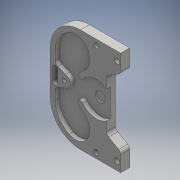
# Autodesk Inventor part: Kompliteringsbit
Saved by Autodesk Inventor 2016 (Build 200138000, 138)
## iProperties
Created: 2017-03-24
Part Number: Kompliteringsbit
Material: Generic
Document SubType Name: Modeling
Designer: 16wise
Density: 1 g/cm^3
Appearance: Default
Author: 16wise
Autodesk Inventor part; units mm, degrees
ref_plane "YZ Plane" through (0, 0, 0) normal (1, 0, 0) x (0, 1, 0)
ref_plane "XZ Plane" through (0, 0, 0) normal (0, 1, 0) x (-1, 0, 0)
ref_plane "XY Plane" through (0, 0, 0) normal (0, 0, 1) x (1, 0, 0)
sketch "Sketch2" plane through (0, 0, 0) normal (0, 1, 0) x (-1, 0, 0)
  line L0 (-51.5, -51.5) -> (51.5, -51.5)
  line L1 (51.5, -51.5) -> (51.5, 51.5)
  line L2 (51.5, 51.5) -> (-51.5, 51.5)
  line L3 (-51.5, 51.5) -> (-51.5, -51.5)
  line L4 (-51.5, -51.5) -> (51.5, 51.5) construction
  line L5 (51.5, -51.5) -> (-51.5, 51.5) construction
  point P0 (0, 0)
  dimension "d6" = 103
  dimension "d7" = 103
  constraints: 12 end point, 2 midpoint, 2 parallel, 1 horizontal, 1 perpendicular
  measures "d6" distance of L2.end L1.end
  measures "d7" distance of L1.end L0.end
extrude "Extrusion2" add sketch "Sketch2" along normal blind 9
fillet "Fillet3" radius 30 1 edges at (-51.5, 4.5, -51.5)
fillet "Fillet4" radius 30 1 edges at (51.5, 4.5, -51.5)
fillet "Fillet5" radius 30 1 edges at (-51.5, 4.5, 51.5)
sketch "Sketch3" plane through (0, 0, 0) normal (0, -1, 0) x (1, 0, 0)
  line L0 (51.5, 51.5) -> (51.5, -21.5) projected
  line L1 (21.5, -51.5) -> (-21.5, -51.5) projected
  line L2 (51.5, 51.5) -> (18.5, 51.5)
  line L3 (18.5, 51.5) -> (18.5, -51.5)
  line L4 (18.5, -51.5) -> (51.5, -51.5)
  line L5 (51.5, -51.5) -> (51.5, 51.5)
  point P0 (0, 0)
  dimension "d13" = 33
  constraints: 8 end point, 2 parallel, 1 horizontal, 1 perpendicular, 1 point on line
  measures "d13" distance of L4.end L3.end
extrude "Extrusion3" cut sketch "Sketch3" against normal blind 9
sketch "Sketch4" plane through (0, 0, 0) normal (0, -1, 0) x (1, 0, 0)
  line L0 (-21.5, 51.5) -> (18.5, 51.5) projected
  line L1 (18.5, 51.5) -> (18.5, 25.5)
  line L2 (18.5, 51.5) -> (18.5, -51.5) projected
  line L3 (18.5, -51.5) -> (18.5, -25.5)
  line L4 (18.5, 25.5) -> (4.5, 25.5)
  line L5 (4.5, 25.5) -> (4.5, -25.5)
  line L6 (4.5, -25.5) -> (18.5, -25.5)
  line L7 (18.5, -25.5) -> (18.5, 25.5)
  point P0 (0, 0)
  dimension "d16" = 26
  dimension "d17" = 26
  dimension "d18" = 14
  constraints: 12 end point, 2 parallel, 2 point on line, 1 horizontal, 1 perpendicular
  measures "d16" distance of L0.end L1.end
  measures "d17" distance of L2.end L3.end
  measures "d18" distance of L6.end L5.end
extrude "Extrusion4" cut sketch "Sketch4" against normal blind 9
sketch "Sketch5" plane through (0, 0, 0) normal (0, -1, 0) x (1, 0, 0)
  line L0 (18.5, 51.5) -> (18.5, 33.5)
  line L1 (18.5, 25.5) -> (18.5, 51.5) projected
  line L2 (4.5, 25.5) -> (4.5, -25.5) projected
  line L3 (18.5, 33.5) -> (4.5, 25.5)
  line L4 (18.5, 25.5) -> (4.5, 25.5) projected
  line L5 (4.5, 25.5) -> (18.5, 25.5)
  line L6 (18.5, 25.5) -> (18.5, 33.5)
  line L7 (18.5, -51.5) -> (-21.5, -51.5) projected
  line L8 (18.5, -51.5) -> (18.5, -33.5)
  line L9 (18.5, -25.5) -> (18.5, -51.5) projected
  line L10 (18.5, -33.5) -> (4.5, -25.5)
  line L11 (4.5, -25.5) -> (18.5, -25.5)
  line L12 (18.5, -25.5) -> (18.5, -33.5)
  point P0 (0, 0)
  dimension "d21" = 18
  dimension "d22" = 18
  constraints: 16 end point, 3 collinear, 2 point on line, 1 perpendicular
  measures "d21" distance of L0.start L0.end
  measures "d22" distance of L7.start L8.end
extrude "Extrusion5" cut sketch "Sketch5" against normal blind 9
fillet "Fillet6" radius 4 4 edges at (4.5, 4.5, 25.5) (18.5, 4.5, 33.5) (18.5, 4.5, -33.5) (4.5, 4.5, -25.5)
sketch "Sketch6" plane through (0, 0, 0) normal (0, -1, 0) x (1, 0, 0)
  line L0 (-21.5, 51.5) -> (18.5, 51.5) projected
  line L1 (18.5, 51.5) -> (18.5, 43)
  line L2 (18.5, 35.8213) -> (18.5, 51.5) projected
  line L3 (18.5, 43) -> (15, 43)
  circle A0 centre (15, 43) radius 2.5
  line L4 (18.5, -51.5) -> (-21.5, -51.5) projected
  line L5 (18.5, -51.5) -> (18.5, -43)
  line L6 (18.5, -35.8213) -> (18.5, -51.5) projected
  line L7 (18.5, -43) -> (15, -43)
  circle A1 centre (15, -43) radius 2.5
  line L8 (18.5, -51.5) -> (-5.5, -51.5)
  line L9 (-5.5, -51.5) -> (-5.5, -46)
  circle A2 centre (-5.5, -46) radius 2.5
  line L10 (18.5, 51.5) -> (-5.5, 51.5)
  line L11 (-5.5, 51.5) -> (-5.5, 46)
  circle A3 centre (-5.5, 46) radius 2.5
  point P0 (0, 0)
  dimension "d26" = 8.5
  dimension "d27" = 3.5
  dimension "d28" = 5
  dimension "d29" = 8.5
  dimension "d30" = 5
  dimension "d31" = 24
  dimension "d32" = 5.5
  dimension "d33" = 5
  dimension "d34" = 5.5
  constraints: 16 end point, 4 centre point, 4 coincident, 4 point on line, 2 horizontal, 2 perpendicular
  measures "d26" distance of L0.end L1.end
  measures "d27" distance of L1.end L3.end
  measures "d28" diameter of A0
  measures "d29" distance of L4.start L5.end
  measures "d30" diameter of A1
  measures "d31" distance of L4.start L8.end
  measures "d32" distance of L8.end L9.end
  measures "d33" diameter of A2
  measures "d34" distance of L10.end L11.end
extrude "Extrusion6" cut sketch "Sketch6" against normal blind 9
sketch "Sketch7" plane through (0, 0, 0) normal (0, -1, 0) x (1, 0, 0)
  line L0 (4.5, 23.1787) -> (4.5, -23.1787) projected
  line L1 (4.5, 0) -> (-5.5, 0)
  circle A0 centre (-5.5, 0) radius 5
  circle A1 centre (-5.5, 0) radius 17
  point P0 (0, 0)
  dimension "d37" = 10
  dimension "d38" = 34
  constraints: 2 centre point, 2 coincident, 2 end point, 1 horizontal, 1 midpoint
  measures "d37" distance of L1.start L1.end
  measures "d38" diameter of A1
extrude "Extrusion7" cut sketch "Sketch7" against normal blind 4
sketch "Sketch8" plane through (-5.5, 0, 0) normal (0, -1, 0) x (1, 0, 0)
  circle A0 centre (0, 0) radius 5
  point P0 (5.5, 0)
  constraints: 1 centre point
extrude "Extrusion8" cut sketch "Sketch8" against normal blind 5
sketch "Sketch9" plane through (0, 0, 0) normal (0, -1, 0) x (1, 0, 0)
  line L0 (-21.5, 51.5) -> (18.5, 51.5) projected
  arc A0 (-21.5, 51.5) -> (-51.5, 21.5) centre (-21.5, 21.5) ccw projected
  line L1 (-51.5, -21.5) -> (-51.5, 21.5) projected
  arc A1 (-51.5, -21.5) -> (-21.5, -51.5) centre (-21.5, -21.5) ccw projected
  line L2 (18.5, -51.5) -> (-21.5, -51.5) projected
  line L3 (18.5, -46.5) -> (-21.5, -46.5)
  arc A2 (-46.5, -21.5) -> (-21.5, -46.5) centre (-21.5, -21.5) ccw
  line L4 (-46.5, -21.5) -> (-46.5, 21.5)
  arc A3 (-21.5, 46.5) -> (-46.5, 21.5) centre (-21.5, 21.5) ccw
  line L5 (-21.5, 46.5) -> (18.5, 46.5)
  arc A4 (4.5, 13.7477) -> (4.5, -13.7477) centre (-5.5, 0) ccw projected
  arc A5 (7.4412, 17.7912) -> (7.4412, -17.7912) centre (-5.5, 0) ccw
  arc A6 (-18.6225, 17.6579) -> (-25.2059, 46.2238) centre (-28.1661, 30.5) ccw
  arc A7 (-25.2059, -46.2238) -> (-18.6225, -17.6579) centre (-28.1661, -30.5) ccw
  arc A8 (5.9706, 15.7695) -> (5.9706, -15.7695) centre (-5.5, 0) ccw
  circle A9 centre (-5.5, 0) radius 5 projected
  line L6 (-5.5, 0) -> (-21.5, 11.1467)
  line L7 (-5.5, 0) -> (-21.5, -11.1467)
  circle A10 centre (-21.5, 11.1467) radius 2.5
  circle A11 centre (-21.5, -11.1467) radius 2.5
  point P0 (0, 0)
  dimension "d43" = 5
  dimension "d44" = 5
  dimension "d45" = 32
  dimension "d46" = 32
  dimension "d47" = 2.5
  constraints: 18 point on circle, 10 end point, 8 centre point, 5 tangent, 2 coincident, 4 other
  measures "d43" radial gap between concentric circles of A0 A3
  measures "d44" radial gap between concentric circles of A4 A5
  measures "d45" diameter of A6
  measures "d46" diameter of A7
  measures "d47" radial gap between concentric circles of A4 A8
extrude "Extrusion9" cut sketch "Sketch9" against normal blind 4 contours L4 A3 A6 A5 A7 A2
sketch "Sketch10" plane through (0, 0, 0) normal (0, -1, 0) x (1, 0, 0)
  arc A0 (4.5, 13.7477) -> (4.5, -13.7477) centre (-5.5, 0) ccw projected
  line L0 (-5.5, 0) -> (-21.1252, 11.6663)
  line L1 (-5.5, 0) -> (-21.1252, -11.6663)
  line L2 (-21.1252, 11.6663) -> (-23.1284, 13.162)
  arc A1 (-18.6225, 17.6579) -> (-18.6225, -17.6579) centre (-5.5, 0) ccw projected
  line L3 (-21.1252, -11.6663) -> (-23.1284, -13.162)
  arc A2 (-19.122, 10.1707) -> (-19.122, -10.1707) centre (-5.5, 0) ccw
  arc A3 (7.4412, 17.7912) -> (7.4412, -17.7912) centre (-5.5, 0) ccw
  arc A4 (-19.122, 10.1707) -> (-19.122, -10.1707) centre (-5.5, 0) ccw
  point P0 (0, 0)
  dimension "d52" = 5
  dimension "d53" = 5
  constraints: 8 end point, 8 point on circle, 3 centre point, 2 point on line
  measures "d52" radial gap between concentric circles of A0 A3
  measures "d53" radial gap between concentric circles of A1 A4
extrude "Extrusion10" cut sketch "Sketch10" against normal blind 4 contours A0 L1 L3 A1 L2 L0
sketch "Sketch11" plane through (0, 4, 0) normal (0, -1, 0) x (1, 0, 0)
  line L0 (-23.1284, 13.162) -> (-19.122, 10.1707) projected
  circle A0 centre (-21.1252, 11.6663) radius 2.5
  line L1 (-19.122, -10.1707) -> (-23.1284, -13.162) projected
  circle A1 centre (-21.1252, -11.6663) radius 2.5
  point P0 (0, 0)
  dimension "d56" = 5
  dimension "d57" = 5
  constraints: 2 centre point, 2 midpoint
  measures "d56" diameter of A0
  measures "d57" diameter of A1
extrude "Extrusion11" add sketch "Sketch11" along normal blind 4
fillet "Fillet7" radius 14 1 edges at (-25.2059, 2, -46.2238)
fillet "Fillet8" radius 14 1 edges at (-25.2059, 2, 46.2238)
sketch "Sketch12" plane through (0, 4, 0) normal (0, -1, 0) x (1, 0, 0)
  line L0 (-46.5, -21.5) -> (-46.5, 21.5) projected
  line L1 (-46.5, 0) -> (-31.5, 0)
  line L2 (-31.5, 0) -> (-31.5, 10)
  line L3 (-31.5, 10) -> (-46.5, 10)
  line L4 (-46.5, 10) -> (-46.5, 0)
  line L5 (-46.5, 0) -> (-31.5, 0)
  line L6 (-31.5, 0) -> (-31.5, -10)
  line L7 (-31.5, -10) -> (-46.5, -10)
  line L8 (-46.5, -10) -> (-46.5, 0)
  arc A0 (-36.4424, -5.9061) -> (-36.1425, 5.8444) centre (-37.5, 0) ccw
  line L9 (-46.5, 10) -> (-46.5, -10)
  line L10 (-46.5, -10) -> (-36.4424, -5.9061)
  line L11 (-46.5, 10) -> (-36.1425, 5.8444)
  line L12 (-46.5, 10) -> (-46.5, -10)
  point P0 (0, 0)
  dimension "d62" = 15
  dimension "d63" = 10
  dimension "d64" = 15
  dimension "d65" = 10
  dimension "d66" = 12
  constraints: 24 end point, 4 parallel, 2 horizontal, 2 perpendicular, 2 point on circle, 1 centre point, 1 collinear, 1 midpoint, 1 point on line, 1 tangent, 1 vertical
  measures "d62" distance of L3.end L2.end
  measures "d63" distance of L2.end L1.end
  measures "d64" distance of L6.end L7.end
  measures "d65" distance of L5.end L6.end
  measures "d66" diameter of A0
extrude "Extrusion12" add sketch "Sketch12" along normal blind 4 contours L0 L1 A0 L10 | L0 L11 A0 L1
fillet "Fillet9" radius 4 2 edges at (-46.5, 2, -10) (-46.5, 2, 10)
sketch "Sketch13" plane through (0, 0, 0) normal (0, -1, 0) x (1, 0, 0)
  arc A0 (-36.4424, -5.9061) -> (-36.1425, 5.8444) centre (-37.5, 0) ccw projected
  arc A1 (-37.1475, -1.9687) -> (-37.0475, 1.9481) centre (-37.5, 0) ccw
  circle A2 centre (-37.5, 0) radius 2
  line L0 (-51.5, -21.5) -> (-51.5, 21.5) projected
  line L1 (-51.5, 0) -> (-46.5, 0)
  line L2 (-46.5, 3.5) -> (-46.5, 6)
  line L3 (-46.5, -3.5) -> (-46.5, -6)
  arc A3 (-44, 6) -> (-49, 6) centre (-46.5, 6) ccw
  arc A4 (-49, -6) -> (-44, -6) centre (-46.5, -6) ccw
  line L4 (-44, -6) -> (-44, 6)
  line L5 (-49, 6) -> (-49, -6)
  point P0 (0, 0)
  dimension "d70" = 4
  dimension "d71" = 5
  dimension "d72" = 6
  dimension "d73" = 6
  dimension "d74" = 5
  dimension "d75" = 5
  constraints: 10 end point, 8 point on circle, 4 centre point, 3 coincident, 3 vertical, 2 tangent, 1 horizontal, 1 midpoint
  measures "d70" radial gap between concentric circles of A0 A1
  measures "d71" distance of L1.start L1.end
  measures "d72" distance of L1.end L2.end
  measures "d73" distance of L1.end L3.end
  measures "d74" diameter of A3
  measures "d75" diameter of A4
extrude "Extrusion13" cut sketch "Sketch13" against normal blind 9
body "Solid2"
